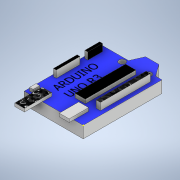
# Autodesk Inventor part: arduino now
Saved by Autodesk Inventor 2021 (Build 250183000, 183)
## iProperties
Created: 2021-07-14
Part Number: arduino now
Material: Generic
Document SubType Name: Modeling
Designer: Dell
Density: 1 g/cm^3
Appearance: Default
Author: Dell
Autodesk Inventor part; units mm, degrees
ref_plane "YZ Plane" through (0, 0, 0) normal (1, 0, 0) x (0, 1, 0)
ref_plane "XZ Plane" through (0, 0, 0) normal (0, 1, 0) x (-1, 0, 0)
ref_plane "XY Plane" through (0, 0, 0) normal (0, 0, 1) x (1, 0, 0)
sketch "Sketch1" plane through (0, 0, 0) normal (0, 1, 0) x (-1, 0, 0)
  line L0 (0, 0) -> (0, -100)
  line L1 (0, 0) -> (75, 0)
  line L2 (75, 0) -> (75, -100)
  line L3 (75, -100) -> (42.4007, -100)
  line L4 (42.4007, -100) -> (35.8215, -115.0757)
  line L5 (35.8215, -115.0757) -> (18.8427, -115.0757)
  line L6 (18.8427, -115.0757) -> (8.0187, -100)
  line L7 (8.0187, -100) -> (0, -100)
  dimension "d0" = 100
  dimension "d1" = 75
  constraints: 16 end point, 2 vertical, 1 collinear, 1 horizontal, 1 parallel, 1 perpendicular, 1 point on line
  measures "d0" distance of L0.start L0.end
  measures "d1" distance of L0.start L1.end
extrude "Extrusion1" add sketch "Sketch1" along normal blind 15
sketch "Sketch2" plane through (0, 15, 0) normal (0, 1, 0) x (1, 0, 0)
  line L0 (-72.4361, 34.6384) -> (-68.8116, 34.6384)
  line L1 (-68.8116, 34.6384) -> (-68.8116, 64.722)
  line L2 (-68.8116, 64.722) -> (-72.4361, 64.722)
  line L3 (-72.4361, 64.722) -> (-72.4361, 34.6384)
  line L4 (-72.4361, 74.6291) -> (-68.8116, 74.6291)
  line L5 (-68.8116, 74.6291) -> (-68.8116, 93.3558)
  line L6 (-68.8116, 93.3558) -> (-72.4361, 93.3558)
  line L7 (-72.4361, 93.3558) -> (-72.4361, 74.6291)
  point P0 (0, 0)
  constraints: 16 end point, 4 parallel, 2 horizontal, 2 perpendicular, 2 point on line
extrude "Extrusion2" add sketch "Sketch2" along normal blind 9
sketch "Sketch3" plane through (0, 15, 0) normal (0, 1, 0) x (1, 0, 0)
  line L0 (-10.6109, 27.0955) -> (-5.1141, 27.0955)
  line L1 (-5.1141, 27.0955) -> (-5.1141, 90.5375)
  line L2 (-5.1141, 90.5375) -> (-10.6109, 90.5375)
  line L3 (-10.6109, 90.5375) -> (-10.6109, 27.0955)
  point P0 (0, 0)
  constraints: 8 end point, 2 parallel, 1 horizontal, 1 perpendicular
extrude "Extrusion3" add sketch "Sketch3" along normal blind 9
sketch "Sketch4" plane through (0, 15, 0) normal (0, 1, 0) x (1, 0, 0)
  line L0 (-24.5308, -5.8613) -> (-11.9398, -5.8613)
  line L1 (-11.9398, -5.8613) -> (-11.9398, 18.8865)
  line L2 (-11.9398, 18.8865) -> (-24.5308, 18.8865)
  line L3 (-24.5308, 18.8865) -> (-24.5308, -5.8613)
  line L4 (-64.0405, -22.7941) -> (-51.8837, -22.7941)
  line L5 (-51.8837, -22.7941) -> (-51.8837, 11.9398)
  line L6 (-51.8837, 11.9398) -> (-64.0405, 11.9398)
  line L7 (-64.0405, 11.9398) -> (-64.0405, -22.7941)
  line L8 (-71.8556, 3.6905) -> (-67.0797, 3.6905)
  line L9 (-67.0797, 3.6905) -> (-67.0797, 11.9398)
  line L10 (-67.0797, 11.9398) -> (-71.8556, 11.9398)
  line L11 (-71.8556, 11.9398) -> (-71.8556, 3.6905)
  point P0 (0, 0)
  constraints: 24 end point, 6 parallel, 3 horizontal, 3 perpendicular, 1 point on line
extrude "Extrusion4" add sketch "Sketch4" along normal blind 4
sketch "Sketch5" plane through (0, 15, 0) normal (0, 1, 0) x (1, 0, 0)
  line L0 (-35.3851, 24.965) -> (-22.3599, 24.965)
  line L1 (-22.3599, 24.965) -> (-22.3599, 89.2226)
  line L2 (-22.3599, 89.2226) -> (-35.3851, 89.2226)
  line L3 (-35.3851, 89.2226) -> (-35.3851, 24.965)
  point P0 (0, 0)
  constraints: 8 end point, 2 parallel, 1 horizontal, 1 perpendicular
extrude "Extrusion5" add sketch "Sketch5" along normal blind 5
sketch "Sketch6" plane through (0, 15, 0) normal (0, 1, 0) x (1, 0, 0)
  line L0 (-62.9909, 21.9257) -> (-62.9909, 90.0836) construction
  line L1 (-62.9909, 90.0836) -> (-37.1661, 90.0836) construction
  line L2 (-37.1661, 90.0836) -> (-37.1661, 21.9257) construction
  line L3 (-37.1661, 21.9257) -> (-62.9909, 21.9257) construction
  point P0 (0, 0)
  constraints: 2 other
sketch "Sketch7" plane through (0, 15, 0) normal (0, 1, 0) x (1, 0, 0)
  point P0 (0, 0)
  point P1 (-14.8096, 97.5183)
  point P2 (-45.0522, 94.6629)
hole "Hole1" at (-14.8096, 15, -97.5183) at (-45.0522, 15, -94.6629) direction (0, -1, 0) diameter 8 end through all
body "Solid1"
